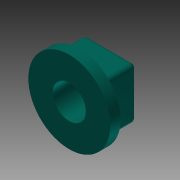
# Autodesk Inventor part: Free Spinning Gear Insert
Saved by Autodesk Inventor 2013 (Build 170138000, 138)
## iProperties
Category: Motion
Company: Autodesk Inc.
Created: 2012-02-22
Part Number: Free Spinning Gear Insert
Document SubType Name: Modeling
Designer: Autodesk Inc.
Density: 1.42 g/cm^3
Material: Acetal Resin, White
Catalog Web Link: http://www.vexrobotics.com/products/accessories/motion/276-2250.html#
Vendor: VEX
Mass: 0.260623 g
Surface Area: 3.24322 cm^2
Volume: 0.183538 cm^3
Author: Autodesk Inc.
Autodesk Inventor part; units mm, degrees
ref_plane "YZ Plane" through (0, 0, 0) normal (1, 0, 0) x (0, 1, 0)
ref_plane "XZ Plane" through (0, 0, 0) normal (0, 1, 0) x (-1, 0, 0)
ref_plane "XY Plane" through (0, 0, 0) normal (0, 0, 1) x (1, 0, 0)
sketch "Sketch1" plane through (0, 0, 0) normal (0, 0, 1) x (1, 0, 0)
  circle A0 centre (0, 0) radius 5.0165
  dimension "d0" = 10.033
  constraints: 1 centre point, 1 coincident
  measures "d0" diameter of A0
extrude "Extrusion1" add sketch "Sketch1" against normal blind 1.27
sketch "Sketch2" plane through (0, 0, -1.27) normal (0, 0, -1) x (-1, 0, 0)
  circle A0 centre (0, 0) radius 5.0165 projected
  line L0 (-3.1496, -3.1496) -> (3.1496, -3.1496)
  line L1 (3.1496, -3.1496) -> (3.1496, 3.1496)
  line L2 (3.1496, 3.1496) -> (-3.1496, 3.1496)
  line L3 (-3.1496, 3.1496) -> (-3.1496, -3.1496)
  point P0 (0, 3.1496)
  point P1 (-3.1496, 0)
  dimension "d3" = 6.2992
  constraints: 8 end point, 2 midpoint, 2 parallel, 2 perpendicular, 1 horizontal, 1 horizontal alignment, 1 vertical alignment
  measures "d3" distance of L1.end L2.end
extrude "Extrusion2" add sketch "Sketch2" along normal blind 3.81 contours L3 L2 L1 L0
fillet "Fillet1" radius 0.508 8 edges at (3.1496, 3.1496, -3.175) (-3.1496, 3.1496, -3.175) (-3.1496, -3.1496, -3.175) (3.1496, -3.1496, -3.175) (3.1496, 0, -5.08) (0, 3.1496, -5.08) (-3.1496, 0, -5.08) (0, -3.1496, -5.08)
sketch "Sketch3" plane through (0, 0, 0) normal (0, 0, 1) x (1, 0, 0)
  circle A0 centre (0, 0) radius 5.0165 projected
hole "Hole1" at (0, 0, 0) direction (0, 0, -1) diameter 4.064 end through all
body "Solid1"
